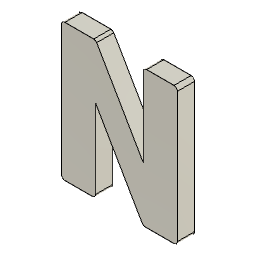
North (Autodesk Fusion 360 design; units mm, degrees)
Autodesk Fusion 360 part; units mm, degrees
sketch "Sketch1" plane through (0, 0, 0) normal (0, 1, 0) x (1, 0, 0)
  line L0 (0, -1.27) -> (0, -49.53)
  line L1 (1.27, -50.8) -> (11.9668, -50.8)
  line L2 (13.0666, -50.165) -> (30.3061, -20.3053)
  line L3 (30.3061, -20.3053) -> (30.3061, -49.5153)
  line L4 (31.5761, -50.7853) -> (41.7361, -50.7853)
  line L5 (43.0061, -49.5153) -> (43.0061, -1.2553)
  line L6 (41.7361, 0.0147) -> (31.0393, 0.0147)
  line L7 (29.9395, -0.6203) -> (12.7, -30.48)
  line L8 (12.7, -30.48) -> (12.7, -1.27)
  line L9 (11.43, 0) -> (1.27, 0)
  arc A0 (0, -49.53) -> (1.27, -50.8) centre (1.27, -49.53) ccw
  arc A1 (1.27, 0) -> (0, -1.27) centre (1.27, -1.27) ccw
  arc A2 (12.7, -1.27) -> (11.43, 0) centre (11.43, -1.27) ccw
  arc A3 (11.9668, -50.8) -> (13.0666, -50.165) centre (11.9668, -49.53) ccw
  arc A4 (30.3061, -49.5153) -> (31.5761, -50.7853) centre (31.5761, -49.5153) ccw
  arc A5 (41.7361, -50.7853) -> (43.0061, -49.5153) centre (41.7361, -49.5153) ccw
  arc A6 (43.0061, -1.2553) -> (41.7361, 0.0147) centre (41.7361, -1.2553) ccw
  arc A7 (31.0393, 0.0147) -> (29.9395, -0.6203) centre (31.0393, -1.2553) ccw
  point P0 (0, -50.8)
  point P1 (12.7, -50.8)
  point P2 (30.3061, -50.7853)
  point P3 (43.0061, -50.7853)
  point P4 (43.0061, 0.0147)
  point P5 (30.3061, 0.0147)
  point P6 (12.7, 0)
  dimension "d6" = 12.7
  dimension "d7" = 12.7
  dimension "d8" = 12.7
  dimension "d9" = 12.7
  dimension "d11" = 30
  dimension "d12" = 30
  dimension "d13" = 50.8
  dimension "d14" = 50.8
  dimension "d15" = 1.27
  dimension "d16" = 1.27
  dimension "d19" = 43.0061
  constraint vertical L0
  constraint perpendicular L0 L1
  constraint vertical L3
  constraint perpendicular L3 L4
  constraint perpendicular L4 L5
  constraint perpendicular L5 L6
  constraint vertical L8
  constraint perpendicular L0 L9
  constraint coincident P0 L0
  constraint coincident P0 L1
  constraint tangent L0 A0
  constraint tangent L1 A0
  constraint coincident origin L0
  constraint coincident origin L9
  constraint tangent L0 A1
  constraint tangent L9 A1
  constraint coincident P6 L8
  constraint coincident P6 L9
  constraint tangent L8 A2
  constraint tangent L9 A2
  constraint equal A1 A2
  constraint coincident P1 L1
  constraint coincident P1 L2
  constraint tangent L1 A3
  constraint tangent L2 A3
  constraint equal A1 A3
  constraint coincident P2 L3
  constraint coincident P2 L4
  constraint tangent L3 A4
  constraint tangent L4 A4
  constraint equal A1 A4
  constraint coincident P3 L4
  constraint coincident P3 L5
  constraint tangent L4 A5
  constraint tangent L5 A5
  constraint equal A1 A5
  constraint coincident P4 L5
  constraint coincident P4 L6
  constraint tangent L5 A6
  constraint tangent L6 A6
  constraint equal A1 A6
  constraint coincident P5 L6
  constraint coincident P5 L7
  constraint tangent L6 A7
  constraint tangent L7 A7
  constraint equal A1 A7
  measures "d6" distance of P0 P1
  measures "d7" distance of P4 P5
  measures "d8" distance of P2 P3
  measures "d9" distance of P6 origin
  measures "d11" angle of L7 L8
  measures "d12" angle of L2 L3
  measures "d13" distance of P3 P4
  measures "d14" distance of origin P0
  measures "d15" radius of A0
  measures "d16" radius of A1
  measures "d19" distance of L0 L5
extrude "Extrude1" add sketch "Sketch1" along normal blind 6.35
